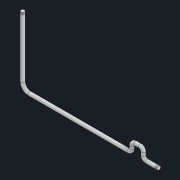
# Autodesk Inventor part: Barra en L
Saved by Autodesk Inventor 2021 (Build 250183000, 183)
## iProperties
Created: 2021-05-06
Part Number: Barra en L
Material: Generic
Document SubType Name: Modeling
Designer: GABRIEL LOL
Density: 1 g/cm^3
Appearance: Default
Author: GABRIEL LOL
Autodesk Inventor part; units mm, degrees
sketch "Sketch1" plane through (0, 0, 0) normal (0, 0, 1) x (1, 0, 0)
  line L0 (0, 6) -> (0, 60)
  line L1 (0, 0) -> (0, 128.6868)
  arc A0 (0, 6) -> (6, 0) centre (6, 6) ccw
  line L2 (120, 0) -> (109.25, 0)
  line L3 (106.25, 3) -> (106.25, 5.75)
  line L4 (103.25, 8.75) -> (99.25, 8.75)
  line L5 (96.25, 5.75) -> (96.25, 3)
  line L6 (93.25, 0) -> (6, 0)
  arc A1 (93.25, 0) -> (96.25, 3) centre (93.25, 3) ccw
  arc A2 (99.25, 8.75) -> (96.25, 5.75) centre (99.25, 5.75) ccw
  arc A3 (106.25, 5.75) -> (103.25, 8.75) centre (103.25, 5.75) ccw
  arc A4 (106.25, 3) -> (109.25, 0) centre (109.25, 3) ccw
  point P0 (106.25, 0)
  point P1 (106.25, 8.75)
  point P2 (96.25, 8.75)
  dimension "d0" = 120
  dimension "d1" = 60
  dimension "d13" = 6
  dimension "d15" = 13.75
  dimension "d16" = 8.75
  dimension "d17" = 10
  dimension "d18" = 3
  constraints: 14 end point, 10 point on circle, 9 tangent, 7 point on line, 5 centre point, 3 equal radius, 3 vertical, 2 horizontal, 2 perpendicular
  measures "d0" distance of L1.start L2.start
  measures "d1" distance of L1.start L0.end
  measures "d13" radius of A0
  measures "d15" distance of L2.start point (106.25, 0)
  measures "d16" distance of point (106.25, 0) point (106.25, 8.75)
  measures "d17" distance of point (106.25, 8.75) point (96.25, 8.75)
  measures "d18" radius of A1
ref_plane "Work Plane1" through (120, 0, 0) normal (1, 0, 0) x (0, 1, 0)
sketch "Sketch2" plane through (120, 0, 0) normal (1, 0, 0) x (0, 1, 0)
  circle A0 centre (0, 0) radius 1.5
  point P0 (0, 0)
  dimension "d2" = 3
  constraints: 1 centre point, 1 coincident
  measures "d2" diameter of A0
sweep "Sweep1" add profiles "Sketch2" path "Sketch1" path curves L2 A4 L3 A3 L4 A2 L5 A1 L6 A0 L0
thread "Thread1"
ref_plane "Work Plane2" through (0, 0, 0) normal (0, 0, 1) x (1, 0, 0)
thread "Thread2"
ref_plane "Work Plane3" through (0, 0, 0) normal (1, 0, 0) x (0, 1, 0)
body "Solid1"
